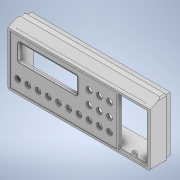
# Autodesk Inventor part: FrontCover
Saved by Autodesk Inventor 2020 (Build 240168000, 168)
## iProperties
Created: 2019-10-18
Part Number: FrontCover
Material: Generic
Document SubType Name: Modeling
Designer: vmiguel
Density: 1 g/cm^3
Appearance: Default
Author: vmiguel
Autodesk Inventor part; units mm, degrees
ref_plane "YZ Plane" through (0, 0, 0) normal (1, 0, 0) x (0, 1, 0)
ref_plane "XZ Plane" through (0, 0, 0) normal (0, 1, 0) x (-1, 0, 0)
ref_plane "XY Plane" through (0, 0, 0) normal (0, 0, 1) x (1, 0, 0)
sketch "Sketch1" plane through (0, 0, 0) normal (0, 0, 1) x (1, 0, 0)
  line L0 (-95.5, 40) -> (95.5, 40)
  line L1 (97.5, 38) -> (97.5, -38)
  line L2 (95.5, -40) -> (-95.5, -40)
  line L3 (-97.5, -38) -> (-97.5, 38)
  line L4 (-97.5, 40) -> (97.5, -40) construction
  line L5 (97.5, 40) -> (-97.5, -40) construction
  arc A0 (-95.5, 40) -> (-97.5, 38) centre (-95.5, 38) ccw
  arc A1 (-97.5, -38) -> (-95.5, -40) centre (-95.5, -38) ccw
  arc A2 (95.5, -40) -> (97.5, -38) centre (95.5, -38) ccw
  arc A3 (97.5, 38) -> (95.5, 40) centre (95.5, 38) ccw
  point P0 (0, 0)
  dimension "d0" = 195
  dimension "d1" = 80
  dimension "d4" = 2
  constraints: 12 end point, 8 point on circle, 8 point on line, 8 tangent, 4 centre point, 3 equal radius, 2 midpoint, 2 parallel, 1 horizontal, 1 perpendicular
  measures "d0" distance of L4.end L5.end
  measures "d1" distance of L5.start L4.end
  measures "d4" radius of A0
extrude "Extrusion1" add sketch "Sketch1" along normal blind 30
sketch "Sketch2" plane through (0, 0, 0) normal (0, 0, -1) x (-1, 0, 0)
  arc A0 (97.5, 38) -> (95.5, 40) centre (95.5, 38) ccw projected
  line L0 (-95.5, 40) -> (95.5, 40) projected
  arc A1 (-95.5, 40) -> (-97.5, 38) centre (-95.5, 38) ccw projected
  line L1 (-97.5, -38) -> (-97.5, 38) projected
  arc A2 (-97.5, -38) -> (-95.5, -40) centre (-95.5, -38) ccw projected
  line L2 (95.5, -40) -> (-95.5, -40) projected
  arc A3 (95.5, -40) -> (97.5, -38) centre (95.5, -38) ccw projected
  line L3 (97.5, 38) -> (97.5, -38) projected
  line L4 (95, 37.5) -> (95, -37.5)
  line L5 (95, -37.5) -> (-95, -37.5)
  line L6 (-95, -37.5) -> (-95, 37.5)
  line L7 (-95, 37.5) -> (95, 37.5)
  point P0 (0, 0)
  dimension "d5" = 2.5
  constraints: 8 end point, 3 other
  measures "d5" distance between parallel lines of L0 L7
extrude "Extrusion2" cut sketch "Sketch2" against normal blind 8
sketch "Sketch3" plane through (97.5, -38, 30) normal (1, 0, 0) x (0, 0, -1)
  line L0 (22, 78) -> (0, 78) projected
  line L1 (0, 78) -> (0, 76) projected
  line L2 (0, 0) -> (0, 76) projected
  line L3 (0, 71) -> (15.0115, 78)
  line L4 (0, 78) -> (15.0115, 78)
  line L5 (0, 71) -> (0, 78)
  point P0 (30, 38)
  dimension "d8" = 25
  dimension "d9" = 7
  constraints: 6 end point, 2 point on line, 1 collinear, 1 perpendicular
  measures "d8" angle of L3 L0
  measures "d9" distance of L3.start L0.end
extrude "Extrusion3" cut sketch "Sketch3" against normal through all
sketch "Sketch4" plane through (0, 0, 30) normal (0, 0, 1) x (1, 0, 0)
  line L0 (97.5, -38) -> (97.5, 33) projected
  line L1 (97.5, 33) -> (-97.5, 33) projected
  line L2 (-95.5, -40) -> (95.5, -40) projected
  line L3 (53.5, 30) -> (93.5, 30)
  line L4 (93.5, 30) -> (93.5, -37)
  line L5 (93.5, -37) -> (53.5, -37)
  line L6 (53.5, -37) -> (53.5, 30)
  point P0 (0, 0)
  dimension "d12" = 3
  dimension "d13" = 4
  dimension "d14" = 3
  dimension "d15" = 40
  constraints: 8 end point, 2 parallel, 1 horizontal, 1 perpendicular
  measures "d12" distance between parallel lines of L1 L3
  measures "d13" distance between parallel lines of L0 L4
  measures "d14" distance between parallel lines of L2 L5
  measures "d15" distance of L3.start L3.end
extrude "Extrusion4" cut sketch "Sketch4" against normal blind 2
sketch "Sketch5" plane through (0, 0, 28) normal (0, 0, 1) x (1, 0, 0)
  line L0 (88.5, 30) -> (88.5, 28)
  line L1 (88.5, 28) -> (58.5, 28)
  line L2 (58.5, 28) -> (58.5, 30)
  line L3 (53.5, -37) -> (53.5, 30) projected
  line L4 (93.5, 30) -> (93.5, -37) projected
  line L5 (58.5, 30) -> (55, 30)
  line L6 (53.5, 30) -> (93.5, 30) projected
  line L7 (55, 30) -> (55, -35)
  line L8 (92, -35) -> (92, 30)
  line L9 (92, 30) -> (88.5, 30)
  line L10 (93.5, -37) -> (53.5, -37) projected
  arc A0 (76.5, -32) -> (70.5, -32) centre (73.5, -32) ccw
  line L11 (70.5, -32) -> (70.5, -35)
  line L12 (76.5, -32) -> (76.5, -35)
  line L13 (55, -35) -> (70.5, -35)
  line L14 (76.5, -35) -> (92, -35)
  point P0 (0, 0)
  point P1 (92, 30)
  dimension "d18" = 5
  dimension "d19" = 5
  dimension "d21" = 2
  dimension "d22" = 1.5
  dimension "d23" = 1.5
  dimension "d25" = 6
  dimension "d26" = 2
  dimension "d27" = 5
  constraints: 22 end point, 7 perpendicular, 2 equal length, 2 horizontal alignment, 2 parallel, 2 point on circle, 2 point on line, 2 tangent, 1 centre point, 1 vertical
  measures "d18" distance between parallel lines of L2 L3
  measures "d19" distance between parallel lines of L4 L0
  measures "d21" distance of L1.end L2.end
  measures "d22" distance between parallel lines of L3 L7
  measures "d23" distance between parallel lines of L4 L8
  measures "d25" diameter of A0
  measures "d26" distance between parallel lines of L10 L13
  measures "d27" distance from line of L10 A0.centre
extrude "Extrusion5" cut sketch "Sketch5" against normal through all contours L6 L8 L14 L12 A0 L11 L13 L7 L5 L2 L1 L0
sketch "Sketch6" plane through (0, 0, 30) normal (0, 0, 1) x (1, 0, 0)
  line L0 (-81.89, 21.59) -> (-4.11, 21.59)
  line L1 (-3.61, 21.09) -> (-3.61, 0.91)
  line L2 (-4.11, 0.41) -> (-81.89, 0.41)
  line L3 (-82.39, 0.91) -> (-82.39, 21.09)
  line L4 (-82.39, 21.59) -> (-3.61, 0.41) construction
  line L5 (-3.61, 21.59) -> (-82.39, 0.41) construction
  line L6 (-87.5, 25) -> (1.5, 25)
  line L7 (1.5, 25) -> (1.5, -3)
  line L8 (1.5, -3) -> (-87.5, -3)
  line L9 (-87.5, -3) -> (-87.5, 25)
  line L10 (-87.5, 25) -> (1.5, -3) construction
  line L11 (1.5, 25) -> (-87.5, -3) construction
  arc A0 (-81.89, 21.59) -> (-82.39, 21.09) centre (-81.89, 21.09) ccw
  arc A1 (-82.39, 0.91) -> (-81.89, 0.41) centre (-81.89, 0.91) ccw
  arc A2 (-4.11, 0.41) -> (-3.61, 0.91) centre (-4.11, 0.91) ccw
  arc A3 (-3.61, 21.09) -> (-4.11, 21.59) centre (-4.11, 21.09) ccw
  line L12 (97.5, 33) -> (-97.5, 33) projected
  line L13 (-97.5, 33) -> (-97.5, -38) projected
  point P0 (0, 0)
  point P1 (-43, 11)
  dimension "d30" = 78.78
  dimension "d31" = 21.18
  dimension "d32" = 89
  dimension "d33" = 28
  dimension "d34" = 0.5
  dimension "d35" = 8
  dimension "d36" = 10
  constraints: 24 end point, 8 point on circle, 8 point on line, 8 tangent, 4 centre point, 4 midpoint, 4 parallel, 3 equal radius, 2 horizontal, 2 perpendicular
  measures "d30" distance of L4.end L5.end
  measures "d31" distance of L5.start L4.end
  measures "d32" distance of L7.end L8.end
  measures "d33" distance of L6.end L7.end
  measures "d34" radius of A0
  measures "d35" distance between parallel lines of L6 L12
  measures "d36" distance between parallel lines of L13 L9
extrude "Extrusion6" cut sketch "Sketch6" against normal through all contours L0 A3 L1 A2 L2 A1 L3 A0
sketch "Sketch7" plane through (0, 0, 30) normal (0, 0, 1) x (1, 0, 0)
  arc A0 (-4.11, 0.41) -> (-3.61, 0.91) centre (-4.11, 0.91) ccw projected
  line L0 (-4.11, 0.41) -> (-81.89, 0.41) projected
  arc A1 (-82.39, 0.91) -> (-81.89, 0.41) centre (-81.89, 0.91) ccw projected
  line L1 (-82.39, 0.91) -> (-82.39, 21.09) projected
  arc A2 (-81.89, 21.59) -> (-82.39, 21.09) centre (-81.89, 21.09) ccw projected
  line L2 (-81.89, 21.59) -> (-4.11, 21.59) projected
  arc A3 (-3.61, 21.09) -> (-4.11, 21.59) centre (-4.11, 21.09) ccw projected
  line L3 (-3.61, 21.09) -> (-3.61, 0.91) projected
  line L4 (93.5, 30) -> (93.5, -37) projected
  line L5 (93.5, -37) -> (53.5, -37) projected
  line L6 (53.5, -37) -> (53.5, 30) projected
  line L7 (53.5, 30) -> (93.5, 30) projected
  line L8 (97.5, 33) -> (-97.5, 33) projected
  line L9 (-97.5, 33) -> (-97.5, -38) projected
  arc A4 (-97.5, -38) -> (-95.5, -40) centre (-95.5, -38) ccw projected
  line L10 (-95.5, -40) -> (95.5, -40) projected
  arc A5 (95.5, -40) -> (97.5, -38) centre (95.5, -38) ccw projected
  line L11 (97.5, -38) -> (97.5, 33) projected
  line L12 (-4.11, 23.59) -> (-81.89, 23.59)
  arc A6 (-81.89, 23.59) -> (-84.39, 21.09) centre (-81.89, 21.09) ccw
  line L13 (-84.39, 21.09) -> (-84.39, 0.91)
  arc A7 (-84.39, 0.91) -> (-81.89, -1.59) centre (-81.89, 0.91) ccw
  line L14 (-81.89, -1.59) -> (-4.11, -1.59)
  arc A8 (-4.11, -1.59) -> (-1.61, 0.91) centre (-4.11, 0.91) ccw
  line L15 (-1.61, 0.91) -> (-1.61, 21.09)
  arc A9 (-1.61, 21.09) -> (-4.11, 23.59) centre (-4.11, 21.09) ccw
  line L16 (-94.5, 30) -> (94.5, 30)
  line L17 (94.5, 30) -> (94.5, -37)
  line L18 (94.5, -37) -> (-94.5, -37)
  line L19 (-94.5, -37) -> (-94.5, 30)
  line L20 (51.5, 30) -> (51.5, -37)
  point P0 (0, 0)
  dimension "d39" = 2
  dimension "d40" = 2
  constraints: 18 end point, 8 point on circle, 4 centre point, 3 point on line, 1 perpendicular, 10 other
  measures "d39" distance between parallel lines of L2 L12
  measures "d40" distance between parallel lines of L6 L20
extrude "Extrusion7" cut sketch "Sketch7" against normal blind 0.4 contours L20 L18 L19 L16
chamfer "Chamfer1" distance 1.4 angle 45 8 edges at (-82.39, 11, 30) (-82.2436, 21.4436, 30) (-43, 21.59, 30) (-3.7564, 21.4436, 30) (-3.61, 11, 30) (-3.7564, 0.5564, 30) (-43, 0.41, 30) (-82.2436, 0.5564, 30)
sketch "Sketch8" plane through (0, 0, 29.6) normal (0, 0, 1) x (1, 0, 0)
  line L0 (-94.5, -37) -> (-94.5, 30) projected
  line L1 (51.5, -37) -> (-94.5, -37) projected
  point P0 (0, 0)
  point P1 (-84.5, -22)
  dimension "d46" = 10
  dimension "d47" = 15
  measures "d46" distance from line of L0 point (-84.5, -22)
  measures "d47" distance from line of L1 point (-84.5, -22)
hole "Hole1" at (-84.5, -22, 29.6) direction (0, 0, -1) diameter 8 end through all
pattern_linear "Rectangular Pattern1" count 10 spacing 14 along (1, 0, 0) of "Hole1"
sketch "Sketch9" plane through (0, 0, 29.6) normal (0, 0, 1) x (1, 0, 0)
  circle A0 centre (41.5, -22) radius 4 projected
  point P0 (0, 0)
  point P1 (41.5, -4)
  dimension "d58" = 18
  constraints: 1 vertical alignment
  measures "d58" distance of A0.centre point (41.5, -4)
hole "Hole2" at (41.5, -4, 29.6) direction (0, 0, -1) diameter 8 end through all
pattern_linear "Rectangular Pattern2" count 3 spacing 14 along (-1, 0, 0) count 2 spacing 18 along (0, 1, 0) of "Hole2"
sketch "Sketch10" plane through (0, 0, 28) normal (0, 0, 1) x (1, 0, 0)
  arc A0 (76.5, -32) -> (70.5, -32) centre (73.5, -32) ccw projected
  point P0 (0, 0)
  constraints: 1 coincident
hole "Hole3" at (73.5, -32, 28) direction (0, 0, -1) diameter 2.013 end through all thread size "M2.5x0.45" class "6H" standard "ANSI Metric M Profile"
sketch "Sketch11" plane through (0, 0, 0) normal (0, 0, -1) x (-1, 0, 0)
  line L0 (95, 37.5) -> (-95, 37.5) projected
  line L1 (-95, 37.5) -> (-95, -37.5) projected
  line L2 (-95, -37.5) -> (95, -37.5) projected
  line L3 (95, -37.5) -> (95, 37.5) projected
  line L4 (-92, -35) -> (-92, 30) projected
  line L5 (-76.5, -35) -> (-92, -35) projected
  line L6 (-92, -35) -> (92, -35)
  line L7 (92, -35) -> (92, 34.5)
  line L8 (92, 34.5) -> (-92, 34.5)
  line L9 (-92, 34.5) -> (-92, -35)
  point P0 (0, 0)
  dimension "d79" = 3
  dimension "d80" = 3
  constraints: 8 end point, 2 parallel, 1 horizontal, 1 perpendicular
  measures "d79" distance between parallel lines of L0 L8
  measures "d80" distance between parallel lines of L3 L7
extrude "Extrusion8" cut sketch "Sketch11" against normal blind 26.5 contours L4 L9 L8 L7 L6 L5
fillet "Fillet1" radius 3 4 edges at (92, 34.5, 13.25) (-92, 34.5, 13.25) (92, -35, 14) (-92, -35, 13.25)
equation "\"d14\" = d12"
equation "\"d19\" = d18"
equation "\"d23\" = d22"
body "Solid1"
